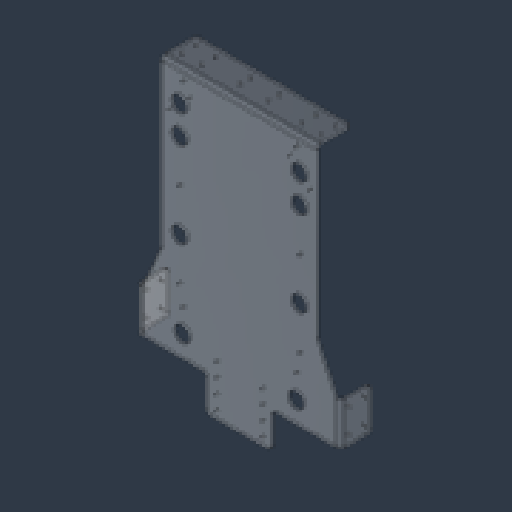
# Autodesk Inventor part: feeder_bottom_plate
Saved by Autodesk Inventor 2024.3 (Build 283343000, 343)
## iProperties
Created: 2025-03-07
Part Number: feeder_bottom_plate
Material: Polycarbonate, Clear
Document SubType Name: Sheet Metal
Designer: marcu
Density: 1.2 g/cm^3
Sheet Metal Rule: Default
Appearance: Polycarbonate - Clear
Mass: 609.438 g
Surface Area: 3304.45 cm^2
Volume: 507.865 cm^3
Author: marcu
Autodesk Inventor part; units mm, degrees
ref_plane "YZ Plane" through (0, 0, 0) normal (1, 0, 0) x (0, 1, 0)
ref_plane "XZ Plane" through (0, 0, 0) normal (0, 1, 0) x (-1, 0, 0)
ref_plane "XY Plane" through (0, 0, 0) normal (0, 0, 1) x (1, 0, 0)
sketch "Sketch1" plane through (0, 0, 0) normal (0, 0, 1) x (1, 0, 0)
  line L0 (139.7, -222.25) -> (-139.7, -222.25)
  line L1 (-139.7, -222.25) -> (-139.7, -69.85) construction
  line L2 (-139.7, 222.25) -> (139.7, 222.25)
  line L3 (139.7, 222.25) -> (139.7, -69.85)
  line L4 (139.7, -222.25) -> (-139.7, 222.25) construction
  line L5 (-139.7, -222.25) -> (139.7, 222.25) construction
  line L6 (-139.7, 222.25) -> (-50.8, 222.25)
  line L7 (-139.7, 209.55) -> (-139.7, 222.25)
  line L8 (139.7, 222.25) -> (50.8, 222.25)
  line L9 (139.7, 209.55) -> (139.7, 222.25)
  line L10 (-57.15, -222.25) -> (57.15, -222.25)
  line L11 (57.15, -222.25) -> (57.15, -311.15)
  line L12 (57.15, -311.15) -> (-57.15, -311.15)
  line L13 (-57.15, -311.15) -> (-57.15, -222.25)
  line L14 (0, 328.93) -> (0, -417.83)
  line L15 (-139.7, -222.25) -> (-152.4, -222.25)
  line L16 (-152.4, -222.25) -> (-152.4, -146.05)
  line L17 (-152.4, -146.05) -> (-139.7, -146.05) construction
  line L18 (-139.7, -146.05) -> (-139.7, -222.25) construction
  line L19 (-152.4, -146.05) -> (-139.7, -69.85)
  line L20 (-139.7, -69.85) -> (-139.7, 222.25)
  line L21 (139.7, -146.05) -> (139.7, -222.25)
  line L22 (139.7, -222.25) -> (152.4, -222.25)
  line L23 (152.4, -222.25) -> (152.4, -146.05)
  line L24 (152.4, -146.05) -> (139.7, -146.05) construction
  line L25 (139.7, -146.05) -> (139.7, -222.25)
  line L26 (152.4, -146.05) -> (139.7, -69.85)
  line L27 (139.7, -69.85) -> (139.7, -222.25) construction
  point P0 (0, 0)
  point P1 (0, -311.15)
  dimension "d0" = 279.4
  dimension "d1" = 444.5
  dimension "d76" = 114.3
  dimension "d77" = 88.9
  dimension "d114" = 12.7
  dimension "d115" = 76.2
  dimension "d117" = 152.4
  measures "d0" distance of L2.start L2.end
  measures "d1" distance of L0.end L2.start
  measures "d76" distance of L11.end L12.end
  measures "d77" distance between parallel lines of L0 L12
  measures "d114" distance of L16.end L17.end
  measures "d115" distance of L15.end L16.end
  measures "d117" distance from line of L0 L1.end
extrude "Plate1" add sketch "Sketch1" along normal blind 4.7625 contours L0 L14 L2 L3 L26 L23 L22 | L0 L15 L16 L19 L20 L7 L2 L14
sketch "Sketch2" plane through (0, 0, 0) normal (0, 0, -1) x (-1, 0, 0)
  line L0 (107.95, 120.65) -> (-107.95, 120.65) construction
  line L1 (-139.7, 222.25) -> (139.7, 222.25) construction
  line L2 (139.7, -222.25) -> (139.7, 222.25) construction
  line L3 (107.95, -32.004) -> (102.6225, -184.565) construction
  line L4 (107.95, -32.004) -> (260.604, -32.004) construction
  line L5 (-107.95, -32.004) -> (-102.6225, -184.565) construction
  line L6 (-107.95, -32.004) -> (44.704, -32.004) construction
  point P0 (0, 0)
  point P1 (0, 120.65)
  point P2 (0, 222.25)
  point P3 (-50.8, 222.25)
  point P4 (50.8, 222.25)
  point P5 (139.7, 209.55)
  point P6 (107.95, 171.704)
  point P7 (-107.95, 171.704)
  dimension "d24" = 9.525
  dimension "d122" = 55.5625
  dimension "d123" = 90
  dimension "d3" = 215.9
  dimension "d4" = 101.6
  dimension "d14" = 152.654
  dimension "d164" = 152.654
  dimension "d165" = 92
  dimension "d166" = 152.654
  dimension "d167" = 88
  dimension "d192" = 51.054
  constraints: 10 end point, 4 coincident, 3 horizontal, 3 vertical alignment, 2 equal length, 2 midpoint, 1 horizontal alignment, 1 vertical, 2 other
  measures "d3" distance of L0.start L0.end
  measures "d4" distance between parallel lines of L0 L1
  measures "d14" distance of point (107.95, 120.65) L3.start
  measures "d164" distance of L3.start L3.end
  measures "d165" angle of L3 L4
  measures "d166" distance of L5.start L5.end
  measures "d167" angle of L5 L6
  measures "d192" distance of point (107.95, 171.704) point (107.95, 120.65)
hole "Hole1" at (-107.95, 120.65, 0) at (107.95, 120.65, 0) at (-107.95, -32.004, 0) at (107.95, -32.004, 0) at (-102.6225, -184.565, 0) at (102.6225, -184.565, 0) at (-107.95, 171.704, 0) at (107.95, 171.704, 0) direction (0, 0, 1) diameter 28.575 end through all
sketch "Sketch3" plane through (139.7, 227.0125, -4.7625) normal (0, 1, 0) x (-1, 0, 0)
  line L0 (279.4, 0) -> (0, 0)
  line L1 (0, 0) -> (0, -53.975)
  line L2 (0, -53.975) -> (279.4, -53.975)
  line L3 (279.4, -53.975) -> (279.4, 0)
  constraints: 6 end point, 1 horizontal, 1 perpendicular, 1 vertical
edge flange "Flange1" height 58.7375 angle 90 thickness 4.7625 bend radius 4.7625 thickness toward (0, 1, 0) relief straight relief width 4.7625 relief depth 2.3813 edges at (0, 222.25, 0) wall of the first edge with corners at (-139.7, 227.0125, -4.7625) (139.7, 227.0125, -4.7625) (139.7, 227.0125, -58.7375) (-139.7, 227.0125, -58.7375)
bend "Bend1"
corner "Corner1"
sketch "Sketch4" plane through (-139.7, 231.775, -58.7375) normal (0, 1, 0) x (1, 0, 0)
  line L0 (0, -53.975) -> (279.4, -53.975) construction
  line L1 (279.4, 0) -> (279.4, -53.975) construction
  line L2 (0, 0) -> (279.4, 0) construction
  line L3 (0, -53.975) -> (0, 0) construction
  point P0 (139.7, -58.7375)
  point P1 (114.3, -34.925)
  point P2 (165.1, -34.925)
  point P3 (114.3, -15.875)
  point P4 (165.1, -15.875)
  dimension "d33" = 114.3
  dimension "d34" = 114.3
  dimension "d37" = 19.05
  dimension "d61" = 15.875
  constraints: 1 horizontal alignment, 1 vertical, 2 other
  measures "d33" distance from line of L3 point (114.3, -34.925)
  measures "d34" distance from line of L1 point (165.1, -34.925)
  measures "d37" distance of point (114.3, -34.925) point (114.3, -15.875)
  measures "d61" distance from line of L2 point (114.3, -15.875)
hole "Hole2" at (-25.4, 231.775, -23.8125) at (25.4, 231.775, -23.8125) at (-25.4, 231.775, -42.8625) at (25.4, 231.775, -42.8625) direction (0, -1, 0) diameter 5.1054 end through all clearance for "Flat Head Machine Screw (82)" size "#10" standard "Ansi Unified Screw Threads"
sketch "Sketch5" plane through (0, 0, 0) normal (0, 0, -1) x (-1, 0, 0)
  circle A0 centre (-107.95, -32.004) radius 14.2875 construction
  circle A1 centre (107.95, -32.004) radius 14.2875 construction
  circle A2 centre (-107.95, 120.65) radius 14.2875 construction
  circle A3 centre (107.95, 120.65) radius 14.2875 construction
  line L0 (-139.7, -69.85) -> (-139.7, 222.25) construction
  line L1 (152.4, -222.25) -> (-152.4, -222.25) construction
  line L2 (-139.7, 222.25) -> (139.7, 222.25) construction
  line L3 (107.95, 120.65) -> (107.95, -32.004) construction
  line L4 (107.95, -32.004) -> (107.95, -184.658) construction
  line L5 (0, 0) -> (0, -25.4) construction
  line L6 (152.4, -146.05) -> (152.4, -222.25) projected
  line L7 (139.7, -69.85) -> (152.4, -146.05) projected
  line L8 (139.7, 222.25) -> (139.7, -69.85) projected
  line L9 (-152.4, -146.05) -> (-139.7, -69.85) projected
  line L10 (-152.4, -222.25) -> (-152.4, -146.05) projected
  point P0 (107.95, -108.331)
  point P1 (107.95, 44.323)
  dimension "d53" = -25.4
  constraints: 6 end point, 2 midpoint, 2 vertical, 1 collinear
  measures "d53" distance of L5.start L5.end
hole "Hole3" at (-107.95, -108.331, 0) at (-107.95, 44.323, 0) direction (0, 0, 1) diameter 5.1054 end through all clearance for "Flat Head Machine Screw (82)" size "#10" standard "Ansi Unified Screw Threads"
sketch "Sketch9" plane through (0, 0, 4.7625) normal (0, 0, 1) x (1, 0, 0)
  circle A0 centre (107.95, 171.704) radius 14.2875 projected
  circle A1 centre (107.95, 171.704) radius 25.4 construction
  line L0 (107.95, 197.104) -> (107.95, 146.304) construction
  line L1 (89.9895, 189.6645) -> (125.9105, 153.7435) construction
  point P0 (0, 0)
  dimension "d193" = 50.8
  dimension "d194" = 45
  constraints: 4 end point, 4 point on circle, 3 coincident, 2 midpoint, 1 centre point, 1 vertical
  measures "d193" diameter of A1
  measures "d194" angle of L0 L1
hole "Hole4" at (125.9105, 153.7435, 4.7625) at (89.9895, 189.6645, 4.7625) direction (0, 0, -1) diameter 4.0386 end through all
mirror "Mirror1" about plane through (0, 0, 0) normal (1, 0, 0) of "Hole4"
mirror "Mirror2" about plane through (0, 0, 0) normal (1, 0, 0) of "Hole3"
sketch "Sketch12" plane through (0, 0, 0) normal (0, 0, -1) x (-1, 0, 0)
  line L0 (152.4, -222.25) -> (152.4, -222.25)
  line L1 (58.7375, -222.25) -> (-58.7375, -222.25)
  line L2 (-58.7375, -222.25) -> (-58.7375, -285.75)
  line L3 (-58.7375, -285.75) -> (58.7375, -285.75)
  line L4 (58.7375, -285.75) -> (58.7375, -222.25)
  line L5 (0, -387.35) -> (0, 323.85) construction
  point P0 (0, 0)
  point P1 (-139.7, -222.25)
  point P2 (139.7, -222.25)
  point P3 (0, -285.75)
  point P4 (0, -222.25)
  dimension "d107" = 63.5
  dimension "d108" = 117.475
  measures "d108" distance between parallel lines of L2 L4
sheet face with bend "Face3" sketch "Sketch12" thickness 4.7625 toward (0, 0, 1) bend radius 4.7625 relief straight relief width 4.7625 relief depth 2.3813
bend "Bend4"
sketch "Sketch13" plane through (-157.1625, -146.05, -4.7625) normal (-1, 0, 0) x (0, -1, 0)
  line L0 (76.2, 0) -> (0, 0)
  line L1 (0, 0) -> (0, -46.0375)
  line L2 (0, -46.0375) -> (76.2, -46.0375)
  line L3 (76.2, -46.0375) -> (76.2, 0)
  constraints: 6 end point, 1 horizontal, 1 perpendicular, 1 vertical
edge flange "Flange3" height 55.5625 angle 90 thickness 4.7625 bend radius 4.7625 thickness toward (-1, 0, 0) relief straight relief width 4.7625 relief depth 2.3813 corner gap 4.7625 corner form 0 edges at (-152.4, -184.15, 0) (152.4, -184.15, 0) wall of the first edge with corners at (-157.1625, -222.25, -4.7625) (-157.1625, -146.05, -4.7625) (-157.1625, -146.05, -50.8) (-157.1625, -222.25, -50.8)
bend "Bend5"
corner "Corner3"
sketch "Sketch14" plane through (-161.925, -222.25, -50.8) normal (-1, 0, 0) x (0, 0, 1)
  line L0 (46.0375, 0) -> (0, 0) projected
  line L1 (55.5625, 0) -> (55.5625, 76.2) projected
  point P0 (50.8, 222.25)
  point P1 (11.1125, 15.875)
  point P2 (11.1125, 60.325)
  point P3 (39.6875, 60.325)
  point P4 (39.6875, 15.875)
  dimension "d130" = 15.875
  dimension "d131" = 44.45
  dimension "d132" = 28.575
  dimension "d133" = 15.875
  constraints: 2 horizontal alignment, 2 vertical alignment
  measures "d130" distance from line of L0 point (11.112, 15.875)
  measures "d131" distance of point (11.112, 60.325) point (11.112, 15.875)
  measures "d132" distance of point (11.112, 15.875) point (39.687, 15.875)
  measures "d133" distance from line of L1 point (39.687, 15.875)
hole "Hole6" at (-161.925, -206.375, -39.6875) at (-161.925, -161.925, -39.6875) at (-161.925, -161.925, -11.1125) at (-161.925, -206.375, -11.1125) direction (1, 0, 0) diameter 5.1054 end through all
sketch "Sketch15" plane through (-139.7, 231.775, -58.7375) normal (0, 1, 0) x (1, 0, 0)
  line L0 (0, -53.975) -> (0, 0) projected
  line L1 (0, 0) -> (279.4, 0) projected
  line L2 (0, -63.5) -> (279.4, -63.5) projected
  line L3 (0, -53.975) -> (279.4, -53.975) projected
  point P0 (139.7, -58.7375)
  point P1 (14.2875, -14.2875)
  point P2 (49.2125, -14.2875)
  point P3 (49.2125, -39.6875)
  point P4 (14.2875, -39.6875)
  dimension "d141" = 14.2875
  dimension "d143" = 25.4
  dimension "d144" = 34.925
  dimension "d153" = 14.2875
  constraints: 2 horizontal alignment, 2 vertical alignment
  measures "d141" distance from line of L0 point (14.287, -14.288)
  measures "d143" distance of point (14.287, -39.688) point (14.287, -14.288)
  measures "d144" distance of point (49.212, -14.288) point (14.287, -14.288)
  measures "d153" distance from line of L3 point (14.287, -39.688)
hole "Hole7" at (-125.4125, 231.775, -44.45) at (-90.4875, 231.775, -44.45) at (-90.4875, 231.775, -19.05) at (-125.4125, 231.775, -19.05) direction (0, -1, 0) diameter 5.1054 end through all
mirror "Mirror3" about plane through (0, 0, 0) normal (1, 0, 0) of "Hole7"
sketch "Sketch16" plane through (0, 0, 4.7625) normal (0, 0, 1) x (1, 0, 0)
  line L0 (-41.275, -273.05) -> (-41.275, -171.45) construction
  line L1 (-58.7375, -285.75) -> (-58.7375, -222.25) construction
  line L2 (58.7375, -285.75) -> (-58.7375, -285.75) projected
  line L3 (-41.275, -273.05) -> (-41.275, -222.25) construction
  line L4 (-41.275, -222.25) -> (-41.275, -171.45) construction
  point P0 (0, 0)
  point P1 (-41.275, -196.85)
  point P2 (-41.275, -247.65)
  dimension "d154" = 17.4625
  dimension "d155" = 12.7
  dimension "d156" = 101.6
  constraints: 6 end point, 3 midpoint, 2 coincident, 1 collinear, 1 vertical
  measures "d154" distance between parallel lines of L1 L0
  measures "d155" distance from line of L2 L0.start
  measures "d156" distance of L0.start L0.end
hole "Hole8" at (-41.275, -196.85, 4.7625) at (-41.275, -222.25, 4.7625) at (-41.275, -247.65, 4.7625) at (-41.275, -273.05, 4.7625) direction (0, 0, -1) diameter 4.5 depth 4.7625 tip angle 118
mirror "Mirror4" about plane through (0, 0, 0) normal (1, 0, 0) of "Hole8"
sketch "Sketch18" plane through (0, 0, 0) normal (0, 0, -1) x (-1, 0, 0)
  line L0 (-362.9369, 222.377) -> (362.9369, 222.377) construction
  line L1 (-101.6, 209.677) -> (101.6, 209.677) construction
  line L2 (-139.7, 222.25) -> (139.7, 222.25) construction
  line L3 (101.6, -142.748) -> (-101.6, -142.748) construction
  point P0 (0, 0)
  point P1 (0, 209.677)
  point P2 (0, 222.25)
  dimension "d181" = 203.2
  dimension "d182" = 12.7
  dimension "d183" = 203.2
  dimension "d184" = 352.425
  constraints: 6 end point, 2 horizontal, 2 midpoint, 2 vertical alignment, 1 parallel, 2 other
  measures "d181" distance of L1.start L1.end
  measures "d182" distance between parallel lines of L0 L1
  measures "d183" distance of L3.start L3.end
  measures "d184" distance of L1.end L3.start
hole "Hole9" at (101.6, 209.677, 0) at (-101.6, 209.677, 0) at (-101.6, -142.748, 0) at (101.6, -142.748, 0) direction (0, 0, 1) diameter 5.1054 end through all clearance for "Flat Head Machine Screw (82)" size "#10" standard "Ansi Unified Screw Threads"
fillet "Corner Round1" radius 6.35 12 edges at (-139.7, 229.3938, -58.7375) (139.7, 229.3938, -58.7375) (-159.5438, -222.25, -50.8) (-159.5438, -146.05, -50.8) (159.5437, -222.25, -50.8) (159.5437, -146.05, -50.8) (-139.7, -69.85, 2.3813) (139.7, -69.85, 2.3813) (-58.7375, -222.25, 2.3813) (-58.7375, -285.75, 2.3813) (58.7375, -285.75, 2.3813) (58.7375, -222.25, 2.3813)
equation "\"d24\" = MinimumRemnant"
equation "\"d10\" = Thickness"
equation "\"d34\" = d33"
equation "\"d92\" = Thickness"
equation "\"d133\" = d130"
equation "\"d139\" = Thickness"
equation "\"d153\" = d141"
equation "\"d162\" = Thickness"
equation "\"d190\" = Thickness"
equation "\"d2\" = Thickness"
equation "\"d22\" = BendReliefWidth"
equation "\"d23\" = BendReliefDepth"
equation "\"d25\" = TransitionRadius"
equation "\"d28\" = BendRadius"
equation "\"d29\" = CornerReliefSize"
equation "\"d30\" = GapSize"
equation "\"d31\" = JacobiRadiusSize"
equation "\"d109\" = BendRadius"
equation "\"d110\" = BendReliefWidth"
equation "\"d112\" = MinimumRemnant"
equation "\"d111\" = BendReliefDepth"
equation "\"d113\" = TransitionRadius"
equation "\"d118\" = BendReliefWidth"
equation "\"d119\" = BendReliefDepth"
equation "\"d120\" = MinimumRemnant"
equation "\"d121\" = TransitionRadius"
equation "\"d124\" = BendRadius"
equation "\"d125\" = CornerReliefSize"
equation "\"d126\" = GapSize"
equation "\"d127\" = JacobiRadiusSize"
equation "\"BendRadius\" = Thickness"
equation "\"BendReliefWidth\" = Thickness"
equation "\"BendReliefDepth\" = 0.5 * Thickness"
equation "\"CornerReliefSize\" = 4 * Thickness"
equation "\"MinimumRemnant\" = 2 * Thickness"
equation "\"TransitionRadius\" = BendRadius"
equation "\"JacobiRadiusSize\" = BendRadius"
equation "\"GapSize\" = Thickness"
equation "\"Thickness\" = 4.7625"
body "Solid1"
